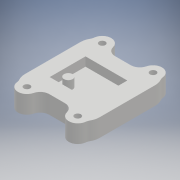
# Autodesk Inventor part: DAQcapsule_v2Bottom
Saved by Autodesk Inventor 2018 (Build 220112000, 112)
## iProperties
Created: 2020-03-10
Part Number: DAQcapsule_v2Bottom
Material: Generic
Document SubType Name: Modeling
Designer: Ivan
Density: 1 g/cm^3
Appearance: Default
Author: Ivan
Autodesk Inventor part; units mm, degrees
ref_plane "YZ Plane" through (0, 0, 0) normal (1, 0, 0) x (0, 1, 0)
ref_plane "XZ Plane" through (0, 0, 0) normal (0, 1, 0) x (-1, 0, 0)
ref_plane "XY Plane" through (0, 0, 0) normal (0, 0, 1) x (1, 0, 0)
sketch "Sketch1" plane through (0, 0, 0) normal (0, 0, 1) x (1, 0, 0)
  line L0 (-12.5, 11) -> (12.5, 11)
  line L1 (12.5, 11) -> (12.5, -11)
  line L2 (12.5, -11) -> (-12.5, -11)
  line L3 (-12.5, -11) -> (-12.5, 11)
  point P0 (0, 0)
  point P1 (0, 11)
  point P2 (12.5, 0)
  dimension "d0" = 25
  dimension "d1" = 22
  constraints: 8 end point, 2 midpoint, 2 parallel, 1 horizontal, 1 horizontal alignment, 1 perpendicular, 1 vertical alignment
  measures "d0" distance of L0.start L0.end
  measures "d1" distance of L0.end L1.end
extrude "Extrusion1" add sketch "Sketch1" along normal blind 3
sketch "Sketch2" plane through (0, 0, 0) normal (0, 0, -1) x (-1, 0, 0)
  circle A0 centre (8.5, -12.6) radius 3
  line L0 (-12.5, -11) -> (-12.5, 11) construction
  line L1 (12.5, -11) -> (-12.5, -11) construction
  circle A1 centre (8.5, -12.6) radius 1.05
  line L2 (12.5, -11) -> (-12.5, -11) construction
  line L3 (0, -11) -> (0, 11) construction
  line L4 (-12.5, 11) -> (12.5, 11) construction
  line L5 (12.5, 11) -> (12.5, -11) construction
  line L6 (12.5, 0) -> (-12.5, 0) construction
  circle A2 centre (-8.5, -12.6) radius 3
  circle A3 centre (-8.5, -12.6) radius 1.05
  circle A4 centre (8.5, 12.6) radius 3
  circle A5 centre (8.5, 12.6) radius 1.05
  circle A6 centre (-8.5, 12.6) radius 3
  circle A7 centre (-8.5, 12.6) radius 1.05
  point P0 (0, 0)
  dimension "d4" = 6
  dimension "d5" = 2.1
  dimension "d6" = 4
  dimension "d9" = 1.6
  constraints: 8 centre point, 6 end point, 6 symmetric about line, 4 coincident, 4 midpoint, 1 perpendicular, 6 other
  measures "d4" diameter of A0
  measures "d5" diameter of A1
  measures "d6" horizontal distance of L1.start A0.centre
  measures "d9" distance from line of A0.centre L1
extrude "Extrusion2" add sketch "Sketch2" against normal blind 6
sketch "Sketch3" plane through (0, 0, 3) normal (0, 0, 1) x (1, 0, 0)
  line L0 (12.5, 11) -> (12.5, -11) projected
  line L1 (-12.5, 11) -> (12.5, 11)
  line L2 (12.5, 11) -> (12.5, 6)
  line L3 (12.5, 6) -> (-12.5, 6)
  line L4 (-12.5, 6) -> (-12.5, 11)
  line L5 (12.5, 6) -> (7.5, 6)
  line L6 (7.5, 6) -> (7.5, -11)
  line L7 (7.5, -11) -> (12.5, -11)
  line L8 (12.5, -11) -> (12.5, 6)
  line L9 (-12.5, 11) -> (-12.5, -11) projected
  line L10 (7.5, -11) -> (-12.5, -11)
  line L11 (-12.5, -11) -> (-12.5, -6)
  line L12 (-12.5, -6) -> (7.5, -6)
  line L13 (7.5, -6) -> (7.5, -11)
  line L14 (-12.5, -6) -> (-7.5, -6)
  line L15 (-7.5, -6) -> (-7.5, 6)
  line L16 (-7.5, 6) -> (-12.5, 6)
  line L17 (-12.5, 6) -> (-12.5, -6)
  point P0 (0, 0)
  dimension "d10" = 5
  dimension "d11" = 5
  dimension "d12" = 5
  dimension "d13" = 5
  constraints: 32 end point, 8 parallel, 4 horizontal, 4 perpendicular, 3 point on line
  measures "d10" distance of L1.end L2.end
  measures "d11" distance of L7.end L6.end
  measures "d12" distance of L10.end L11.end
  measures "d13" distance of L16.end L15.end
sketch "Sketch4" plane through (0, 0, 3) normal (0, 0, 1) x (1, 0, 0)
  circle A0 centre (-4.5, -2.75) radius 1.45
  line L0 (-12.5, 11) -> (-12.5, -11) projected
  line L1 (-5.9623, -11) -> (5.9623, -11) projected
  point P0 (0, 0)
  dimension "d14" = 2.9
  dimension "d15" = 8
  dimension "d16" = 8.25
  constraints: 1 centre point
  measures "d14" diameter of A0
  measures "d15" distance from line of L0 A0.centre
  measures "d16" distance from line of L1 A0.centre
extrude "Extrusion3" add sketch "Sketch4" along normal blind 3
sketch "Sketch5" plane through (0, 0, 3) normal (0, 0, 1) x (1, 0, 0)
  circle A0 centre (-4.5, -2.75) radius 1.45 construction
  line L0 (4, 5.5) -> (6, 5.5)
  line L1 (6, 5.5) -> (6, -5.5)
  line L2 (6, -5.5) -> (4, -5.5)
  line L3 (4, -5.5) -> (4, 5.5)
  point P0 (0, 0)
  dimension "d19" = 2
  dimension "d20" = 11
  dimension "d21" = 8.5
  dimension "d22" = 2.75
  constraints: 8 end point, 2 parallel, 1 horizontal, 1 perpendicular
  measures "d19" distance of L1.end L2.end
  measures "d20" distance of L0.end L1.end
  measures "d21" distance from line of A0.centre L3
  measures "d22" distance from line of A0.centre L2
extrude "Extrusion4" cut sketch "Sketch5" against normal blind 0.75
extrude "Extrusion5" add sketch "Sketch3" along normal blind 3 contours L0 L3 L4 L1 | L0 L7 L6 L3 | L3 L15 L12 L9 | L10 L9 L12 L6
ref_plane "Work Plane1" through (0, 0, 1) normal (0, 0, -1) x (-1, 0, 0)
sketch "Sketch7" plane through (0, 0, 1) normal (0, 0, -1) x (-1, 0, 0)
  circle A0 centre (-8.475, -12.61) radius 1.05
  point P0 (0, 0)
  dimension "d31" = 2.1
  constraints: 1 centre point, 1 coincident
  measures "d31" diameter of A0
sketch "Sketch8" plane through (0, 0, 0) normal (0, 0, -1) x (-1, 0, 0)
  circle A0 centre (-8.475, -12.61) radius 1.8
  point P0 (0, 0)
  dimension "d32" = 3.6
  constraints: 1 centre point, 1 coincident
  measures "d32" diameter of A0
loft "Loft1" cut profiles "Sketch8", "Sketch7"
mirror "Mirror1" about plane through (0, 0, 0) normal (1, 0, 0) of "Loft1"
mirror "Mirror2" about plane through (0, 0, 0) normal (0, 1, 0) of "Loft1", "Mirror1"
fillet "Fillet1" radius 3 8 edges at (11.0377, -11, 3) (5.9623, -11, 3) (-5.9623, -11, 3) (-11.0377, -11, 3) (11.0377, 11, 3) (5.9623, 11, 3) (-11.0377, 11, 3) (-5.9623, 11, 3)
fillet "Fillet2" radius 5 4 edges at (12.5, 11, 3) (-12.5, 11, 3) (-12.5, -11, 3) (12.5, -11, 3)
sketch "Sketch9" plane through (7.5, -6, 3) normal (-1, 0, 0) x (0, 0, 1)
  line L0 (0, 0) -> (3, 0) projected
  line L1 (3, 12) -> (3, 0) projected
  line L2 (0, 12) -> (3, 12) projected
  line L3 (0, 0) -> (0, 12) projected
  point P0 (-3, 6)
extrude "Extrusion7" add sketch "Sketch9" along normal blind 1
equation "\"d10\" = d13"
equation "\"d11\" = d13"
equation "\"d12\" = d13"
body "Solid1"
